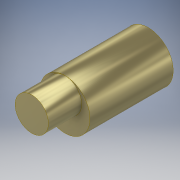
# Autodesk Inventor part: connector
Saved by Autodesk Inventor 2019 (Build 230136000, 136)
## iProperties
Created: 2018-06-15
Part Number: connector
Material: Generic
Document SubType Name: Modeling
Designer: daniel
Density: 1 g/cm^3
Appearance: Default
Author: daniel
Autodesk Inventor part; units mm, degrees
ref_plane "YZ Plane" through (0, 0, 0) normal (1, 0, 0) x (0, 1, 0)
ref_plane "XZ Plane" through (0, 0, 0) normal (0, 1, 0) x (-1, 0, 0)
ref_plane "XY Plane" through (0, 0, 0) normal (0, 0, 1) x (1, 0, 0)
sketch "Sketch1" plane through (0, 0, 0) normal (0, 0, 1) x (1, 0, 0)
  circle A0 centre (0, 0) radius 3.75
  dimension "d4" = 7.5
  constraints: 1 centre point, 1 coincident
  measures "d4" diameter of A0
extrude "Extrusion1" add sketch "Sketch1" along normal blind 12.5
sketch "Sketch2" plane through (0, 0, 12.5) normal (0, 0, 1) x (1, 0, 0)
  circle A0 centre (0, 1.25) radius 2.5
  line L0 (0, 6.75) -> (0, -5.5) projected
  circle A1 centre (0, 0) radius 3.75 projected
  point P0 (0, 3.75)
  dimension "d5" = 5
  constraints: 2 point on line, 2 vertical alignment, 1 coincident, 3 other
extrude "Extrusion2" add sketch "Sketch2" along normal blind 5 contours A0 L0 | L0 A0
body "Solid1"
